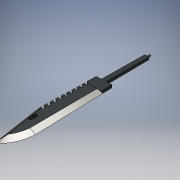
# Autodesk Inventor part: Main
Saved by Autodesk Inventor 2018 (Build 220112000, 112)
## iProperties
Created: 2020-11-24
Part Number: Main
Material: Všeobecné
Document SubType Name: Modeling
Designer: Jozko Mrkvicka
Density: 1 g/cm^3
Appearance: Výchozí
Author: Jozko Mrkvicka
Autodesk Inventor part; units mm, degrees
ref_plane "YZ Plane" through (0, 0, 0) normal (1, 0, 0) x (0, 1, 0)
ref_plane "XZ Plane" through (0, 0, 0) normal (0, 1, 0) x (-1, 0, 0)
ref_plane "XY Plane" through (0, 0, 0) normal (0, 0, 1) x (1, 0, 0)
ref_plane "Pracovní rovina3" through (0, 156, 0) normal (0, 1, 0) x (1, 0, 0)
sketch "sketch_Knife" plane through (0, 156, 0) normal (0, 1, 0) x (1, 0, 0)
  line L0 (4.85, 76.2339) -> (-11.35, 0)
  arc A0 (-32.85, 41.2339) -> (-11.35, 0) centre (28.5011, 47.0012) ccw
  line L1 (-32.85, 41.2339) -> (-32.85, 157.5)
  line L2 (-30, 157.5) -> (-30, 180)
  line L3 (-32.85, 157.5) -> (-30, 157.5)
  line L4 (-30, 180) -> (-19, 180)
  line L5 (-9, 180) -> (2, 180)
  line L6 (-19, 180) -> (-19, 291)
  line L7 (-9, 291) -> (-9, 180)
  line L8 (2, 180) -> (2, 157.5)
  arc A1 (-5.6271, 50.4174) -> (-4.85, 52) centre (-6.85, 52) ccw
  line L9 (-4.85, 52) -> (-4.85, 60)
  arc A2 (-4.85, 60) -> (-6.85, 62) centre (-6.85, 60) ccw
  line L10 (-6.85, 62) -> (-8.85, 62)
  arc A3 (-8.85, 62) -> (-10.85, 60) centre (-8.85, 60) ccw
  line L11 (-10.85, 60) -> (-10.85, 52)
  arc A4 (-10.85, 52) -> (-8.85, 50) centre (-8.85, 52) ccw
  line L12 (-8.85, 50) -> (-6.85, 50)
  arc A5 (-6.85, 50) -> (-5.6271, 50.4174) centre (-6.85, 52) ccw
  line L13 (4.85, 76.2339) -> (4.85, 157.5)
  line L14 (-9, 291) -> (-19, 291)
  line L15 (4.85, 157.5) -> (2, 157.5)
  dimension "bladeWidth" = 37.7
  dimension "bladeLength" = 157.5
  dimension "handleLength" = 111
  dimension "lenght" = 22.5
  dimension "holeWidth" = 6
  dimension "holeLength" = 12
  dimension "handleWidth" = 10
  dimension "width" = 32
  dimension "width2" = 11
  dimension "width3" = 2.85
  dimension "knifeHoleVerticalOffset" = 22
  constraints: 32 end point, 12 point on circle, 6 centre point, 1 horizontal, 1 horizontal alignment, 1 parallel, 1 perpendicular, 1 point on line
  measures "bladeWidth" distance between parallel lines of L1 L13
  measures "bladeLength" distance from line of L0.end L3
  measures "handleLength" distance of L4.end L6.end
  measures "lenght" distance of L2.start L2.end
  measures "holeWidth" distance between parallel lines of L11 L9
  measures "holeLength" distance between parallel lines of L10 L12
  measures "handleWidth" distance of L7.start L6.end
  measures "width" distance between parallel lines of L2 L8
  measures "width2" distance of L5.start L5.end
  measures "width3" distance of L13.end L8.end
  measures "knifeHoleVerticalOffset" distance between parallel lines of L1 L11
extrude "Knife" add sketch "sketch_Knife" along normal blind 6
ref_plane "Pracovní rovina4" through (-30, 156, -157.5) normal (0, 0, -1) x (-1, 0, 0)
split body "Rozdělit1" result two bodies by plane through (-30, 156, -157.5) normal (0, 0, -1) first body at (-12.3333, 156.5, -217)
chamfer "Zkosení103" distance 11 distance2 3 1 edges at (-32.85, 156, -99.3669) measured on face at (-32.35, 156, -99.3669)
chamfer "Zkosení104" distance 11 distance2 3 1 edges at (-16.9636, 156, -5.4057) measured on face at (-16.5947, 156, -5.7432)
chamfer "Zkosení105" distance 11 distance2 3 1 edges at (-32.85, 162, -99.3669) measured on face at (-32.35, 162, -99.3669)
chamfer "Zkosení106" distance 11 distance2 3 1 edges at (-16.9636, 162, -5.4057) measured on face at (-16.5947, 162, -5.7432)
chamfer "Zkosení107" distance 5 distance2 3 1 edges at (-1.9077, 156, -44.4333) measured on face at (-2.3968, 156, -44.5372)
chamfer "Zkosení108" distance 7 distance2 2 1 edges at (4.85, 156, -128.8941) measured on face at (4.35, 156, -128.8941)
chamfer "Zkosení109" distance 5 distance2 3 1 edges at (-1.9078, 162, -44.4333) measured on face at (-2.3968, 162, -44.5372)
chamfer "Zkosení110" distance 7 distance2 2 1 edges at (4.85, 162, -128.8941) measured on face at (4.35, 162, -128.8941)
chamfer "Zkosení111" distance 2 distance2 1 1 edges at (4.85, 158, -120.876) measured on face at (4.3692, 157.8626, -120.876)
chamfer "Zkosení112" distance 2 distance2 1 1 edges at (4.85, 160, -120.876) measured on face at (4.3692, 160.1374, -120.876)
sketch "sketch_Teeth" plane through (0, 156, 0) normal (0, -1, 0) x (1, 0, 0)
  line L0 (4.85, -157.5) -> (4.85, -76.2339) projected
  arc A0 (-1.15, -73.7679) -> (-3.15, -77.2321) centre (-2.15, -75.5) ccw
  line L1 (-3.15, -77.2321) -> (3.7936, -81.2409)
  line L2 (-1.15, -73.7679) -> (4.85, -77.2321)
  line L3 (4.85, -77.2321) -> (4.85, -87.2321)
  line L4 (3.7936, -81.2409) -> (4.85, -87.2321)
  line L5 (4.85, -87.2321) -> (4.85, -97.2321)
  line L6 (3.7936, -91.2409) -> (4.85, -97.2321)
  line L7 (-3.15, -87.2321) -> (3.7936, -91.2409)
  line L8 (-1.15, -83.7679) -> (4.85, -87.2321)
  arc A1 (-1.15, -83.7679) -> (-3.15, -87.2321) centre (-2.15, -85.5) ccw
  line L9 (4.85, -97.2321) -> (4.85, -107.2321)
  line L10 (3.7936, -101.2409) -> (4.85, -107.2321)
  line L11 (-3.15, -97.2321) -> (3.7936, -101.2409)
  line L12 (-1.15, -93.7679) -> (4.85, -97.2321)
  arc A2 (-1.15, -93.7679) -> (-3.15, -97.2321) centre (-2.15, -95.5) ccw
  line L13 (4.85, -107.2321) -> (4.85, -117.2321)
  line L14 (3.7936, -111.2409) -> (4.85, -117.2321)
  line L15 (-3.15, -107.2321) -> (3.7936, -111.2409)
  line L16 (-1.15, -103.7679) -> (4.85, -107.2321)
  arc A3 (-1.15, -103.7679) -> (-3.15, -107.2321) centre (-2.15, -105.5) ccw
  line L17 (4.85, -117.2321) -> (4.85, -127.2321)
  line L18 (3.7936, -121.2409) -> (4.85, -127.2321)
  line L19 (-3.15, -117.2321) -> (3.7936, -121.2409)
  line L20 (-1.15, -113.7679) -> (4.85, -117.2321)
  arc A4 (-1.15, -113.7679) -> (-3.15, -117.2321) centre (-2.15, -115.5) ccw
  line L21 (4.85, -127.2321) -> (4.85, -137.2321)
  line L22 (3.7936, -131.2409) -> (4.85, -137.2321)
  line L23 (-3.15, -127.2321) -> (3.7936, -131.2409)
  line L24 (-1.15, -123.7679) -> (4.85, -127.2321)
  arc A5 (-1.15, -123.7679) -> (-3.15, -127.2321) centre (-2.15, -125.5) ccw
  line L25 (4.85, -137.2321) -> (4.85, -147.2321)
  line L26 (3.7936, -141.2409) -> (4.85, -147.2321)
  line L27 (-3.15, -137.2321) -> (3.7936, -141.2409)
  line L28 (-1.15, -133.7679) -> (4.85, -137.2321)
  arc A6 (-1.15, -133.7679) -> (-3.15, -137.2321) centre (-2.15, -135.5) ccw
  line L29 (4.85, -147.2321) -> (4.85, -157.2321)
  line L30 (3.7936, -151.2409) -> (4.85, -157.2321)
  line L31 (-3.15, -147.2321) -> (3.7936, -151.2409)
  line L32 (-1.15, -143.7679) -> (4.85, -147.2321)
  arc A7 (-1.15, -143.7679) -> (-3.15, -147.2321) centre (-2.15, -145.5) ccw
  line L33 (4.85, -157.2321) -> (4.85, -167.2321)
  line L34 (3.7936, -161.2409) -> (4.85, -167.2321)
  line L35 (-3.15, -157.2321) -> (3.7936, -161.2409)
  line L36 (-1.15, -153.7679) -> (4.85, -157.2321)
  arc A8 (-1.15, -153.7679) -> (-3.15, -157.2321) centre (-2.15, -155.5) ccw
  line L37 (-6.85, -62) -> (-8.85, -62) projected
  point P0 (0, 0)
  dimension "teethRadius_" = 4
  dimension "teethHigh_" = 7
  dimension "teethAngle_" = 60
  dimension "toothAngle2_" = 10
  dimension "toothWidth2_" = 10
  dimension "d471" = 10
  dimension "toothOffset_" = 13.5
  constraints: 72 end point, 18 point on circle, 9 centre point, 2 point on line, 2 tangent, 1 parallel, 1 vertical, 88 other
  measures "teethRadius_" diameter of A0
  measures "teethHigh_" distance from line of L0 A0.centre
  measures "teethAngle_" angle of L0 L1
  measures "toothAngle2_" angle of L0 L4
  measures "toothWidth2_" distance of L3.end L2.end
  measures "d471" distance of L2.end L5.start
  measures "toothOffset_" distance from line of L37 A0.centre
extrude "Teeth" cut sketch "sketch_Teeth" against normal blind 6 bodies 3 2
sketch "sketch_Thread" plane through (-9, 156, -291) normal (0, 0, -1) x (-1, 0, 0)
  circle A0 centre (5, 3) radius 2
  point P0 (-9, -156)
  dimension "knifeThreadDia" = 4
  constraints: 1 centre point
  measures "knifeThreadDia" diameter of A0
extrude "Thread" add sketch "sketch_Thread" along normal blind 10 bodies 2
chamfer "Zkosení113" distance 0.5 angle 45 1 edges at (-12, 159, -301)
thread "Závit3" size "M4x0.7" class "6g" standard "ANSI Metric M Profile" full length
